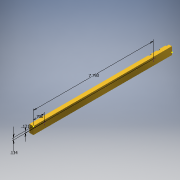
# Autodesk Inventor part: mounting rail 9.0 x.250 x.500-A-sfpcutouts
Saved by Autodesk Inventor 2017 (Build 210142000, 142)
## iProperties
Created: 2014-01-27
Part Number: mounting rail 9.0 x.250 x.500-A-sfpcutouts
Material: Gold
Document SubType Name: Modeling
Designer: rtreacy
Density: 1 g/cm^3
Appearance: Gold - Metal
Author: rtreacy
Autodesk Inventor part; units mm, degrees
ref_plane "YZ Plane" through (0, 0, 0) normal (1, 0, 0) x (0, 1, 0)
ref_plane "XZ Plane" through (0, 0, 0) normal (0, 1, 0) x (-1, 0, 0)
ref_plane "XY Plane" through (0, 0, 0) normal (0, 0, 1) x (1, 0, 0)
sketch "Sketch2" plane through (0, 0, 0) normal (0, 0, 1) x (1, 0, 0)
  line L0 (-8.2799, 8.6846) -> (-1.9299, 8.6846)
  line L1 (-1.9299, 8.6846) -> (-1.9299, -4.0154)
  line L2 (-1.9299, -4.0154) -> (-8.2799, -4.0154)
  line L3 (-8.2799, -4.0154) -> (-8.2799, 8.6846)
  point P0 (0, 0)
  dimension "d3" = 6.35
  dimension "d5" = 12.7
  constraints: 8 end point, 2 parallel, 1 horizontal, 1 perpendicular
  measures "d3" distance of L0.start L0.end
  measures "d5" distance of L2.end L0.start
extrude "Extrusion1" add sketch "Sketch2" along normal blind 228.6
sketch "Sketch3" plane through (-1.9299, -4.0154, 0) normal (1, 0, 0) x (0, 0, -1)
  point P0 (-228.6, 12.7)
  point P1 (0, 4.0154)
  point P2 (-210.82, 9.287)
  point P3 (-30.6578, 9.6266)
  dimension "d8" = 3.413
  dimension "d9" = 17.78
  dimension "d45" = 197.9422
  dimension "d46" = 3.0734
  measures "d8" vertical distance of point (-228.6, 12.7) point (-210.82, 9.287)
  measures "d9" horizontal distance of point (-228.6, 12.7) point (-210.82, 9.287)
  measures "d45" horizontal distance of point (-228.6, 12.7) point (-30.658, 9.627)
  measures "d46" vertical distance of point (-30.658, 9.627) point (-228.6, 12.7)
hole "Hole1" at (-1.9299, 5.2716, 210.82) direction (-1, 0, 0) diameter 1.7018 end through all
pattern_linear "Rectangular Pattern1" count 7 spacing 25.4 along (0, 0, -1) of "Hole1"
sketch "Sketch6" plane through (203.1751, -4.0154, 104.775) normal (0, -1, 0) x (1, 0, 0)
  point P0 (0, 4.0154)
  point P1 (-208.28, -100.965)
  point P2 (-208.28, -46.355)
  point P3 (-211.455, -104.775)
  point P4 (-205.105, -104.775)
  dimension "d68" = 58.42
  dimension "d69" = 3.81
  dimension "d76" = 3.175
  dimension "d77" = 3.175
  measures "d68" vertical distance of point (-208.28, -46.355) point (-211.455, -104.775)
  measures "d69" vertical distance of point (-208.28, -100.965) point (-211.455, -104.775)
  measures "d76" horizontal distance of point (-205.105, -104.775) point (-208.28, -46.355)
  measures "d77" horizontal distance of point (-205.105, -104.775) point (-208.28, -100.965)
hole "Hole2" at (-5.1049, -4.0154, 3.81) direction (0, 1, 0) diameter 1.7018 depth 6.35 tip angle 118
hole "Hole5" at (-5.1049, -4.0154, 58.42) direction (0, 1, 0) diameter 1.7018 depth 6.35 tip angle 118
pattern_linear "Rectangular Pattern5" count 2 spacing 25.4 along (0, 0, 1) of "Hole2"
pattern_linear "Rectangular Pattern6" count 5 spacing 38.1 along (0, 0, 1) of "Hole5"
sketch "Sketch9" plane through (-8.2799, -4.0154, 0) normal (0, -1, 0) x (1, 0, 0)
  line L0 (6.35, 0) -> (6.35, 228.6) projected
  line L1 (0, 0) -> (0, 228.6) projected
  line L2 (6.35, 0) -> (0, 0) projected
  line L3 (0, 0) -> (6.35, 0) projected
  line L4 (6.35, 30.6578) -> (0, 30.6578) construction
  line L5 (6.096, 16.4084) -> (0, 16.4084) construction
  line L6 (0, 0) -> (0, 228.6) construction
  line L7 (6.35, 2.159) -> (0, 2.159) construction
  line L8 (1.524, 32.6898) -> (0, 32.6898)
  line L9 (0, 32.6898) -> (0, 28.6258)
  line L10 (0, 28.6258) -> (1.524, 28.6258)
  line L11 (1.524, 28.6258) -> (1.524, 32.6898)
  line L12 (1.524, 32.6898) -> (0, 28.6258) construction
  line L13 (0, 32.6898) -> (1.524, 28.6258) construction
  line L14 (1.524, 18.4404) -> (0, 18.4404)
  line L15 (0, 18.4404) -> (0, 14.3764)
  line L16 (0, 14.3764) -> (1.524, 14.3764)
  line L17 (1.524, 14.3764) -> (1.524, 18.4404)
  line L18 (1.524, 18.4404) -> (0, 14.3764) construction
  line L19 (0, 18.4404) -> (1.524, 14.3764) construction
  line L20 (1.524, 4.318) -> (0, 4.318)
  line L21 (0, 4.318) -> (0, 0)
  line L22 (0, 0) -> (1.524, 0)
  line L23 (1.524, 0) -> (1.524, 4.318)
  line L24 (1.524, 4.318) -> (0, 0) construction
  line L25 (0, 4.318) -> (1.524, 0) construction
  point P0 (6.35, 4.191)
  point P1 (4.318, 0)
  point P2 (0.762, 30.6578)
  point P3 (0.762, 16.4084)
  point P4 (0.762, 2.159)
  dimension "d78" = 30.6578
  dimension "d93" = 4.064
  dimension "d94" = 1.524
  dimension "d95" = 1.524
  dimension "d96" = 4.064
  dimension "d97" = 1.524
  constraints: 42 end point, 12 point on line, 7 parallel, 6 midpoint, 5 perpendicular, 3 horizontal
  measures "d78" distance from line of L2 L4.start
  measures "d93" distance of L10.end L8.start
  measures "d94" distance of L9.end L10.end
  measures "d95" distance of L15.end L16.end
  measures "d96" distance of L16.end L14.start
  measures "d97" distance of L20.start L20.end
extrude "Extrusion3" cut sketch "Sketch9" against normal through all
body "Solid1"
